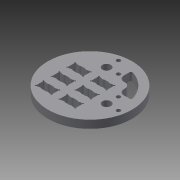
# Autodesk Inventor part: Segment_Small
Saved by Autodesk Inventor 2015 (Build 190159000, 159)
## iProperties
Created: 2012-09-02
Part Number: Segment_Small
Material: Generic
Document SubType Name: Modeling
Designer: ErikEnvy
Density: 1 g/cm^3
Appearance: Default
Author: ErikEnvy
Autodesk Inventor part; units mm, degrees
ref_plane "YZ Plane" through (0, 0, 0) normal (1, 0, 0) x (0, 1, 0)
ref_plane "XZ Plane" through (0, 0, 0) normal (0, 1, 0) x (-1, 0, 0)
ref_plane "XY Plane" through (0, 0, 0) normal (0, 0, 1) x (1, 0, 0)
sketch "Sketch1" plane through (0, 0, 0) normal (0, 0, 1) x (1, 0, 0)
  circle A0 centre (0, 12) radius 1.6
  circle A1 centre (12, 0) radius 1.6
  circle A2 centre (0, 16.5) radius 0.75
  circle A3 centre (16.5, 0) radius 0.75
  arc A4 (-7.25, 7.5) -> (-7.5, 7.25) centre (-7.5, 7.5) ccw
  arc A5 (-6.75, 7.5) -> (-5.25, 7.5) centre (-6, 8.8062) ccw
  arc A6 (-1.5, 7.25) -> (-1.75, 7.5) centre (-1.5, 7.5) ccw
  arc A7 (-3.75, 7.5) -> (-2.25, 7.5) centre (-3, 8.8062) ccw
  arc A8 (-7.5, 4.75) -> (-7.25, 4.5) centre (-7.5, 4.5) ccw
  arc A9 (-5.25, 4.5) -> (-6.75, 4.5) centre (-6, 3.1938) ccw
  arc A10 (-2.25, 4.5) -> (-3.75, 4.5) centre (-3, 3.1938) ccw
  arc A11 (-1.75, 4.5) -> (-1.5, 4.75) centre (-1.5, 4.5) ccw
  line L0 (-1.5, 7.25) -> (-1.5, 4.75)
  line L1 (-1.75, 4.5) -> (-2.25, 4.5)
  line L2 (-2.25, 7.5) -> (-1.75, 7.5)
  line L3 (-3.75, 7.5) -> (-5.25, 7.5)
  line L4 (-5.25, 4.5) -> (-3.75, 4.5)
  line L5 (-7.25, 7.5) -> (-6.75, 7.5)
  line L6 (-7.5, 7.25) -> (-7.5, 4.75)
  line L7 (-6.75, 4.5) -> (-7.25, 4.5)
  arc A12 (1.75, 7.5) -> (1.5, 7.25) centre (1.5, 7.5) ccw
  arc A13 (2.25, 7.5) -> (3.75, 7.5) centre (3, 8.8062) ccw
  arc A14 (5.25, 7.5) -> (6.75, 7.5) centre (6, 8.8062) ccw
  arc A15 (7.5, 7.25) -> (7.25, 7.5) centre (7.5, 7.5) ccw
  arc A16 (6.75, 4.5) -> (5.25, 4.5) centre (6, 3.1938) ccw
  arc A17 (7.25, 4.5) -> (7.5, 4.75) centre (7.5, 4.5) ccw
  arc A18 (3.75, 4.5) -> (2.25, 4.5) centre (3, 3.1938) ccw
  arc A19 (1.5, 4.75) -> (1.75, 4.5) centre (1.5, 4.5) ccw
  line L8 (7.5, 7.25) -> (7.5, 4.75)
  line L9 (7.25, 4.5) -> (6.75, 4.5)
  line L10 (6.75, 7.5) -> (7.25, 7.5)
  line L11 (5.25, 7.5) -> (3.75, 7.5)
  line L12 (3.75, 4.5) -> (5.25, 4.5)
  line L13 (1.75, 7.5) -> (2.25, 7.5)
  line L14 (1.5, 7.25) -> (1.5, 4.75)
  line L15 (2.25, 4.5) -> (1.75, 4.5)
  arc A20 (-7.25, 1.5) -> (-7.5, 1.25) centre (-7.5, 1.5) ccw
  arc A21 (-6.75, 1.5) -> (-5.25, 1.5) centre (-6, 2.8062) ccw
  arc A22 (-3.75, 1.5) -> (-2.25, 1.5) centre (-3, 2.8062) ccw
  arc A23 (-1.5, 1.25) -> (-1.75, 1.5) centre (-1.5, 1.5) ccw
  arc A24 (-2.25, -1.5) -> (-3.75, -1.5) centre (-3, -2.8062) ccw
  arc A25 (-1.75, -1.5) -> (-1.5, -1.25) centre (-1.5, -1.5) ccw
  arc A26 (-5.25, -1.5) -> (-6.75, -1.5) centre (-6, -2.8062) ccw
  arc A27 (-7.5, -1.25) -> (-7.25, -1.5) centre (-7.5, -1.5) ccw
  line L16 (-1.5, 1.25) -> (-1.5, -1.25)
  line L17 (-1.75, -1.5) -> (-2.25, -1.5)
  line L18 (-2.25, 1.5) -> (-1.75, 1.5)
  line L19 (-3.75, 1.5) -> (-5.25, 1.5)
  line L20 (-5.25, -1.5) -> (-3.75, -1.5)
  line L21 (-7.25, 1.5) -> (-6.75, 1.5)
  line L22 (-7.5, 1.25) -> (-7.5, -1.25)
  line L23 (-6.75, -1.5) -> (-7.25, -1.5)
  arc A28 (1.75, 1.5) -> (1.5, 1.25) centre (1.5, 1.5) ccw
  arc A29 (2.25, 1.5) -> (3.75, 1.5) centre (3, 2.8062) ccw
  arc A30 (5.25, 1.5) -> (6.75, 1.5) centre (6, 2.8062) ccw
  arc A31 (7.5, 1.25) -> (7.25, 1.5) centre (7.5, 1.5) ccw
  arc A32 (6.75, -1.5) -> (5.25, -1.5) centre (6, -2.8062) ccw
  arc A33 (7.25, -1.5) -> (7.5, -1.25) centre (7.5, -1.5) ccw
  arc A34 (3.75, -1.5) -> (2.25, -1.5) centre (3, -2.8062) ccw
  arc A35 (1.5, -1.25) -> (1.75, -1.5) centre (1.5, -1.5) ccw
  line L24 (7.5, 1.25) -> (7.5, -1.25)
  line L25 (7.25, -1.5) -> (6.75, -1.5)
  line L26 (6.75, 1.5) -> (7.25, 1.5)
  line L27 (5.25, 1.5) -> (3.75, 1.5)
  line L28 (3.75, -1.5) -> (5.25, -1.5)
  line L29 (1.75, 1.5) -> (2.25, 1.5)
  line L30 (1.5, 1.25) -> (1.5, -1.25)
  line L31 (2.25, -1.5) -> (1.75, -1.5)
  arc A36 (-7.25, -4.5) -> (-7.5, -4.75) centre (-7.5, -4.5) ccw
  arc A37 (-6.75, -4.5) -> (-5.25, -4.5) centre (-6, -3.1938) ccw
  arc A38 (-3.75, -4.5) -> (-2.25, -4.5) centre (-3, -3.1938) ccw
  arc A39 (-1.5, -4.75) -> (-1.75, -4.5) centre (-1.5, -4.5) ccw
  arc A40 (-2.25, -7.5) -> (-3.75, -7.5) centre (-3, -8.8062) ccw
  arc A41 (-1.75, -7.5) -> (-1.5, -7.25) centre (-1.5, -7.5) ccw
  arc A42 (-5.25, -7.5) -> (-6.75, -7.5) centre (-6, -8.8062) ccw
  arc A43 (-7.5, -7.25) -> (-7.25, -7.5) centre (-7.5, -7.5) ccw
  line L32 (-1.5, -4.75) -> (-1.5, -7.25)
  line L33 (-1.75, -7.5) -> (-2.25, -7.5)
  line L34 (-2.25, -4.5) -> (-1.75, -4.5)
  line L35 (-3.75, -4.5) -> (-5.25, -4.5)
  line L36 (-5.25, -7.5) -> (-3.75, -7.5)
  line L37 (-7.25, -4.5) -> (-6.75, -4.5)
  line L38 (-7.5, -4.75) -> (-7.5, -7.25)
  line L39 (-6.75, -7.5) -> (-7.25, -7.5)
  arc A44 (1.75, -4.5) -> (1.5, -4.75) centre (1.5, -4.5) ccw
  arc A45 (2.25, -4.5) -> (3.75, -4.5) centre (3, -3.1938) ccw
  arc A46 (5.25, -4.5) -> (6.75, -4.5) centre (6, -3.1938) ccw
  arc A47 (7.5, -4.75) -> (7.25, -4.5) centre (7.5, -4.5) ccw
  arc A48 (6.75, -7.5) -> (5.25, -7.5) centre (6, -8.8062) ccw
  arc A49 (7.25, -7.5) -> (7.5, -7.25) centre (7.5, -7.5) ccw
  arc A50 (3.75, -7.5) -> (2.25, -7.5) centre (3, -8.8062) ccw
  arc A51 (1.5, -7.25) -> (1.75, -7.5) centre (1.5, -7.5) ccw
  line L40 (7.5, -4.75) -> (7.5, -7.25)
  line L41 (7.25, -7.5) -> (6.75, -7.5)
  line L42 (6.75, -4.5) -> (7.25, -4.5)
  line L43 (5.25, -4.5) -> (3.75, -4.5)
  line L44 (3.75, -7.5) -> (5.25, -7.5)
  line L45 (1.75, -4.5) -> (2.25, -4.5)
  line L46 (1.5, -4.75) -> (1.5, -7.25)
  line L47 (2.25, -7.5) -> (1.75, -7.5)
  circle A52 centre (2.8284, 2.8284) radius 16
  circle A53 centre (4.5, 12) radius 0.75
  circle A54 centre (11.9999, 4.5) radius 0.75
  line L48 (10.5, 8) -> (10.5, 8.5)
  line L49 (8.5, 10.5) -> (8, 10.5)
  line L50 (6, 12.5) -> (6, 14.777)
  line L51 (12.5, 6) -> (14.777, 6)
  arc A55 (15.255, 6.6469) -> (6.6469, 15.255) centre (2.8284, 2.8284) ccw
  arc A56 (10.5, 8.5) -> (8.5, 10.5) centre (8.5, 8.5) ccw
  arc A57 (10.5, 8) -> (12.5, 6) centre (12.5, 8) ccw
  arc A58 (6, 12.5) -> (8, 10.5) centre (8, 12.5) ccw
  arc A59 (6.6469, 15.255) -> (6, 14.777) centre (6.5, 14.777) ccw
  arc A60 (14.777, 6) -> (15.255, 6.6469) centre (14.777, 6.5) ccw
  point P0 (6, 15.4356)
  point P1 (15.4356, 6)
  dimension "d123" = 4.5
  dimension "d124" = 4.5
  dimension "d125" = 4.5
  dimension "d126" = 4.5
  constraints: 110 point on circle, 104 end point, 61 centre point, 10 tangent, 4 perpendicular, 3 equal radius, 3 parallel, 2 point on line, 1 coincident, 1 collinear, 1 vertical, 2 other
  measures "d123" distance of A1.centre A54.centre
  measures "d124" distance of A3.centre A1.centre
  measures "d125" distance of A2.centre A0.centre
  measures "d126" distance of A53.centre A0.centre
extrude "Extrusion1" add sketch "Sketch1" along normal blind 3
body "Solid1"
